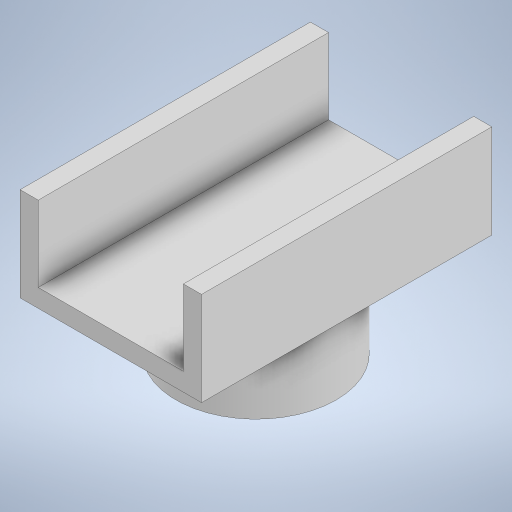
# Autodesk Inventor part: endcap_4mm_2ea_typeB_ver2_onyx_addon
Saved by Autodesk Inventor 2024 (Build 280153000, 153)
## iProperties
Created: 2024-04-25
Part Number: endcap_4mm_2ea_typeB_ver2_onyx_addon
Material: 일반
Document SubType Name: Modeling
Designer: Gihyeok Na
Density: 1 g/cm^3
Appearance: 기본값
Author: Gihyeok Na
Autodesk Inventor part; units mm, degrees
ref_plane "YZ Plane" through (0, 0, 0) normal (1, 0, 0) x (0, 1, 0)
ref_plane "XZ Plane" through (0, 0, 0) normal (0, 1, 0) x (-1, 0, 0)
ref_plane "XY Plane" through (0, 0, 0) normal (0, 0, 1) x (1, 0, 0)
sketch "스케치1" plane through (0, 0, 0) normal (0, 1, 0) x (-1, 0, 0)
  line L0 (-2.4, 4.8) -> (2.4, 4.8)
  line L1 (2.4, 4.8) -> (2.4, -4.8)
  line L2 (2.4, -4.8) -> (-2.4, -4.8)
  line L3 (-2.4, -4.8) -> (-2.4, 4.8)
  line L4 (-2.4, 4.8) -> (2.4, -4.8) construction
  line L5 (2.4, 4.8) -> (-2.4, -4.8) construction
  circle A0 centre (0, 0) radius 2.65
  circle A1 centre (0, 0) radius 1.85
  dimension "d0" = 4.8
  dimension "d1" = 9.6
  dimension "d17" = 5.3
  dimension "d18" = 3.7
  constraints: 12 end point, 2 centre point, 2 coincident, 2 midpoint, 2 parallel, 1 horizontal, 1 perpendicular
  measures "d0" distance of L1.end L2.end
  measures "d1" distance of L0.end L1.end
  measures "d17" diameter of A0
  measures "d18" diameter of A1
extrude "돌출1" add sketch "스케치1" along normal blind 0.6 contours L0 L1 A0 L3 | A0 L1 L3 | A0 L1 L2 L3 | A1
sketch "스케치2" plane through (0, 0, 0) normal (0, -1, 0) x (1, 0, 0)
  line L0 (2.4, -4.8) -> (-2.4, -4.8) projected
  line L1 (2.4, 4.8) -> (2.4, -4.8) projected
  line L2 (-2.4, 4.8) -> (2.4, 4.8) projected
  line L3 (-2.4, -4.8) -> (-2.4, 4.8) projected
  line L4 (2.4, 4.8) -> (3, 4.8)
  line L5 (3, 4.8) -> (3, -4.8)
  line L6 (3, -4.8) -> (2.4, -4.8)
  line L7 (2.4, -4.8) -> (2.4, 4.8)
  line L8 (-2.4, -4.8) -> (-2.4, 4.8) projected
  line L9 (-2.4, 4.8) -> (-3, 4.8)
  line L10 (-3, 4.8) -> (-3, -4.8)
  line L11 (-3, -4.8) -> (-2.4, -4.8)
  line L12 (-2.4, -4.8) -> (-2.4, 4.8)
  point P0 (0, 0)
  dimension "d4" = 0.6
  dimension "d5" = 0.6
  constraints: 16 end point, 4 parallel, 2 horizontal, 2 perpendicular, 1 point on line
  measures "d4" distance of L5.end L6.end
  measures "d5" distance of L11.end L10.end
extrude "돌출2" add sketch "스케치2" against normal blind 3.1 contours L1 L4 L5 L6 | L11 L10 L9 L3
extrude "돌출5" add sketch "스케치1" against normal blind 2.5 contours A0 L1 L3 | L3 A0 | A0 L1
